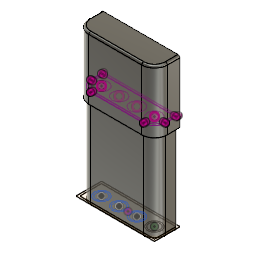
SolderingTipHolder (Autodesk Fusion 360 design; units mm, degrees)
Autodesk Fusion 360 part; units mm, degrees
note: some values were not read from the file. Set by a fixed rule: which sketch regions a step uses.
sketch "Sketch1" plane through (0, 0, 0) normal (0, 0, 1) x (1, 0, 0)
  circle A0 centre (4.5, 0) radius 2.75
  circle A1 centre (-4.5, 0) radius 2.75
  circle A2 centre (13.4322, 0.0419) radius 2.75
  circle A3 centre (-13.5265, 0) radius 2.75
  line L0 (-19, 5.5) -> (19, 5.5)
  line L1 (19, 5.5) -> (19, -5.5)
  line L2 (19, -5.5) -> (-19, -5.5)
  line L3 (-19, -5.5) -> (-19, 5.5)
  circle A4 centre (-4.5, 0) radius 3.5
  circle A5 centre (4.5, 0) radius 3.5
  circle A6 centre (13.4322, 0.0419) radius 3.5
  circle A7 centre (-13.5265, 0) radius 3.5
  line L4 (20, 6.5) -> (20, -6.5)
  line L5 (20, -6.5) -> (-20, -6.5)
  line L6 (-20, -6.5) -> (-20, 6.5)
  line L7 (-20, 6.5) -> (20, 6.5)
  dimension "d1" = 5.5
  dimension "d2" = 5.5
  dimension "d3" = 5.5
  dimension "d4" = 5.5
  dimension "d5" = 7
  dimension "d6" = 7
  dimension "d7" = 7
  dimension "d8" = 7
  dimension "d9" = 5.5
  dimension "d10" = 19
  dimension "d11" = 19
  dimension "d12" = 5.5
  dimension "d23" = 1
  measures "d1" diameter of A0
  measures "d2" diameter of A1
  measures "d3" diameter of A2
  measures "d4" diameter of A3
  measures "d5" diameter of A4
  measures "d6" diameter of A5
  measures "d7" diameter of A6
  measures "d8" diameter of A7
  measures "d9" distance of origin L0
  measures "d10" distance of origin L3
  measures "d11" distance of origin L1
  measures "d12" distance of origin L2
extrude "Extrude1" add sketch "Sketch1" against normal blind 2 contours A0 | A1 | A2 | A3 | L0 L1 L2 L3 | A4 | A5 | A6 | A7 makes body 1
extrude "Extrude2" add sketch "Sketch1" along normal blind 45 contours L0 L1 L2 L3 | A4 | A5 | A6 | A7 bodies 1
sketch "Sketch2" plane through (0, 0, 45) normal (0, 0, 1) x (-1, 0, 0)
  circle A0 centre (13.5265, 0) radius 2.75
  circle A1 centre (-13.4322, -0.0419) radius 2.75
  circle A2 centre (4.5, 0) radius 2.75
  circle A3 centre (-4.5, 0) radius 2.75
  line L0 (-19, 5.5) -> (-19, -5.5)
  line L1 (-19, -5.5) -> (19, -5.5)
  line L2 (19, -5.5) -> (19, 5.5)
  line L3 (19, 5.5) -> (-19, 5.5)
  circle A4 centre (13.5265, 0) radius 3.5
  circle A5 centre (4.5, 0) radius 2.75
  circle A6 centre (13.5265, 0) radius 2.75
  circle A7 centre (13.5265, 0) radius 2.75
  circle A8 centre (4.5, 0) radius 3.5
  line L4 (-19, -5.5) -> (-19, 5.5)
  line L5 (-19, 5.5) -> (19, 5.5)
  line L6 (19, 5.5) -> (19, -5.5)
  line L7 (19, -5.5) -> (-19, -5.5)
  line L8 (19, 5.5) -> (-19, 5.5)
  line L9 (-19, 5.5) -> (19, 5.5)
  circle A9 centre (-13.4322, -0.0419) radius 2.75
  circle A10 centre (-13.4322, -0.0419) radius 2.75
  circle A11 centre (-13.4322, -0.0419) radius 2.75
  circle A12 centre (-13.4322, -0.0419) radius 3.5
  circle A13 centre (-4.5, 0) radius 3.5
extrude "Extrude3" add sketch "Sketch2" along normal blind 3.5 contours L0 L1 L2 L3 L4 L5 L6 L7 L8 L9 bodies 1
fillet "Fillet1" radius 5.5 2 edges at (-19, -5.5, 23.25) (19, -5.5, 23.25) on bodies 1
fillet "Fillet2" radius 1 10 edges at (19, 2.75, -2) (17.3891, -3.8891, -2) (0, -5.5, -2) (-17.3891, -3.8891, -2) (-19, 2.75, -2) (-19, 2.75, 48.5) (-17.3891, -3.8891, 48.5) (0, -5.5, 48.5) (17.3891, -3.8891, 48.5) (19, 2.75, 48.5) on bodies 1
sketch "Sketch3" plane through (0, 0, 48.5) normal (0, 0, 1) x (-1, 0, 0)
  line L0 (18, -5.5) -> (18, 0)
  arc A0 (18, 0) -> (13.5, 4.5) centre (13.5, 0) ccw
  line L1 (13.5, 4.5) -> (-13.5, 4.5)
  arc A1 (-13.5, 4.5) -> (-18, 0) centre (-13.5, 0) ccw
  line L2 (-18, 0) -> (-18, -5.5)
  line L3 (-18, -5.5) -> (18, -5.5)
  circle A2 centre (4.5, 0) radius 3.5
  circle A3 centre (13.5265, 0) radius 3.5
  circle A4 centre (-4.5, 0) radius 3.5
  circle A5 centre (-13.4322, -0.0419) radius 3.5
  line L4 (-20, 6.5) -> (20, 6.5)
  line L5 (-19, 5.5) -> (19, 5.5)
  line L6 (20, 6.5) -> (20, -6.5)
  line L7 (19, 5.5) -> (19, -5.5)
  line L8 (19, -5.5) -> (-19, -5.5)
  line L9 (20, -6.5) -> (-20, -6.5)
  line L10 (-20, -6.5) -> (-20, 6.5)
  line L11 (-19, -5.5) -> (-19, 5.5)
  circle A6 centre (-13.4322, -0.0419) radius 2.75
extrude "Extrude4" add sketch "Sketch3" against normal blind 5 separate body contours L4 L6 L9 L10 makes body 2
move_face "OffsetFaces1" offset 25 1 faces at (6, 6.1667, 48.5) on bodies 2
sketch "Sketch4" plane through (0, 0, 73.5) normal (0, 0, 1) x (-1, 0, 0)
  line L0 (19, -5.5) -> (-19, -5.5)
  line L1 (-19, -5.5) -> (-19, 5.5)
  line L2 (-19, 5.5) -> (19, 5.5)
  line L3 (19, 5.5) -> (19, -5.5)
  line L4 (-20, -6.5) -> (20, -6.5)
  line L5 (20, -6.5) -> (20, 6.5)
  line L6 (20, 6.5) -> (-20, 6.5)
  line L7 (-20, 6.5) -> (-20, -6.5)
  line L8 (20, -6.5) -> (-20, -6.5)
  line L9 (20, 6.5) -> (20, -6.5)
  line L10 (-20, 6.5) -> (20, 6.5)
  line L11 (-20, -6.5) -> (-20, 6.5)
extrude "Extrude5" add sketch "Sketch4" along normal blind 2 contours L0 L1 L2 L3 | L4 L5 L6 L7 L8 L9 L10 L11 bodies 2
fillet "Fillet3" radius 5.5 2 edges at (19, -5.5, 58.5) (-19, -5.5, 58.5) on bodies 2
fillet "Fillet4" radius 6.5 2 edges at (-20, -6.5, 59.5) (20, -6.5, 59.5) on bodies 2
fillet "Fillet5" radius 1 5 edges at (20, 3.25, 75.5) (18.0962, -4.5962, 75.5) (0, -6.5, 75.5) (-18.0962, -4.5962, 75.5) (-20, 3.25, 75.5) on bodies 2
fillet "Fillet6" radius 0.25 10 edges at (20, 3.25, 43.5) (18.0962, -4.5962, 43.5) (0, -6.5, 43.5) (-18.0962, -4.5962, 43.5) (-20, 3.25, 43.5) (-19, 2.75, 43.5) (-17.3891, -3.8891, 43.5) (0, -5.5, 43.5) (17.3891, -3.8891, 43.5) (19, 2.75, 43.5) on bodies 2
sketch "Sketch5" plane through (0, 0, 48.5) normal (0, 0, 1) x (-1, 0, 0)
  line L0 (18, -5.5) -> (18, 0)
  arc A0 (18, 0) -> (13.5, 4.5) centre (13.5, 0) ccw
  line L1 (13.5, 4.5) -> (-13.5, 4.5)
  arc A1 (-13.5, 4.5) -> (-18, 0) centre (-13.5, 0) ccw
  line L2 (-18, 0) -> (-18, -5.5)
  line L3 (-18, -5.5) -> (18, -5.5)
  circle A2 centre (4.5, 0) radius 3.5
  circle A3 centre (13.5265, 0) radius 3.5
  circle A4 centre (-4.5, 0) radius 3.5
  circle A5 centre (-13.4322, -0.0419) radius 3.5
  line L4 (-19, 0) -> (-19, -6.5)
  line L5 (-19, -6.5) -> (19, -6.5)
  line L6 (19, -6.5) -> (19, 0)
  arc A6 (19, 0) -> (13.5, 5.5) centre (13.5, 0) ccw
  line L7 (13.5, 5.5) -> (-13.5, 5.5)
  arc A7 (-13.5, 5.5) -> (-19, 0) centre (-13.5, 0) ccw
  arc A8 (19, 0) -> (13.5, 5.5) centre (13.5, 0) ccw
  line L8 (19, 0) -> (19, -5.5)
  line L9 (19, -5.5) -> (-19, -5.5)
  line L10 (-19, -5.5) -> (-19, 0)
  arc A9 (-13.5, 5.5) -> (-19, 0) centre (-13.5, 0) ccw
  line L11 (-13.5, 5.5) -> (13.5, 5.5)
  line L12 (13.5, 4.5) -> (13.5, 5.5)
  arc A10 (18, 0) -> (13.5, 4.5) centre (13.5, 0) ccw
  line L13 (18, 0) -> (19, 0)
  arc A11 (19, 0) -> (13.5, 5.5) centre (13.5, 0) ccw
  line L14 (-13.5, 4.5) -> (-13.5, 5.5)
  line L15 (-13.5, 4.5) -> (13.5, 4.5)
  line L16 (13.5, 4.5) -> (13.5, 5.5)
  line L17 (13.5, 5.5) -> (-13.5, 5.5)
  line L18 (19, -5.5) -> (18, -5.5)
  line L19 (19, -5.5) -> (19, 0)
  line L20 (18, 0) -> (19, 0)
  line L21 (18, 0) -> (18, -5.5)
  line L22 (-18, -5.5) -> (-19, -5.5)
  line L23 (-18, -5.5) -> (-18, 0)
  line L24 (-18, 0) -> (-19, 0)
  line L25 (-19, 0) -> (-19, -5.5)
  line L26 (-18, 0) -> (-19, 0)
  arc A12 (-13.5, 4.5) -> (-18, 0) centre (-13.5, 0) ccw
  line L27 (-13.5, 4.5) -> (-13.5, 5.5)
  arc A13 (-13.5, 5.5) -> (-19, 0) centre (-13.5, 0) ccw
